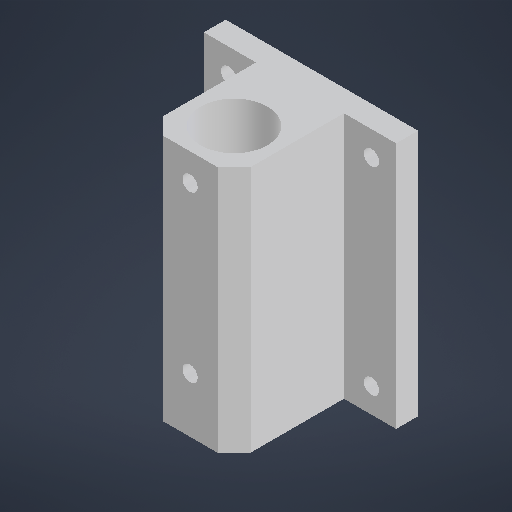
# Autodesk Inventor part: microscope mount
Saved by Autodesk Inventor 2026 (Build 300175050, 175E)
## iProperties
Created: 2025-07-01
Part Number: microscope mount
Material: Generic
Document SubType Name: Modeling
Designer: Tobymegacat
Density: 1 g/cm^3
Appearance: Default
Author: Tobymegacat
Autodesk Inventor part; units mm, degrees
ref_plane "YZ Plane" through (0, 0, 0) normal (1, 0, 0) x (0, 1, 0)
ref_plane "XZ Plane" through (0, 0, 0) normal (0, 1, 0) x (-1, 0, 0)
ref_plane "XY Plane" through (0, 0, 0) normal (0, 0, 1) x (1, 0, 0)
sketch "Sketch1" plane through (0, 0, 0) normal (0, 0, 1) x (1, 0, 0)
  line L0 (-16.3442, 35.2565) -> (18.6558, 35.2565)
  line L1 (18.6558, 35.2565) -> (18.6558, -9.7435)
  line L2 (18.6558, -9.7435) -> (-16.3442, -9.7435)
  line L3 (-16.3442, -9.7435) -> (-16.3442, 35.2565)
  point P0 (0, 0)
  dimension "d0" = 35
  dimension "d1" = 45
  constraints: 8 end point, 2 parallel, 1 horizontal, 1 perpendicular
  measures "d0" distance of L1.end L2.end
  measures "d1" distance between parallel lines of L0 L2
extrude "Extrusion1" add sketch "Sketch1" along normal blind 4
sketch "Sketch2" plane through (0, 0, 4) normal (0, 0, 1) x (1, 0, 0)
  line L0 (-6.8442, -9.7435) -> (9.1558, -9.7435)
  line L1 (9.1558, -9.7435) -> (9.1558, 35.2565)
  line L2 (9.1558, 35.2565) -> (-6.8442, 35.2565)
  line L3 (-6.8442, 35.2565) -> (-6.8442, -9.7435)
  line L4 (-16.3442, -9.7435) -> (18.6558, -9.7435) projected
  line L5 (18.6558, 35.2565) -> (-16.3442, 35.2565) projected
  line L6 (-6.8442, 14.4079) -> (-16.3442, 14.4079)
  line L7 (-16.3442, 35.2565) -> (-16.3442, -9.7435) projected
  line L8 (9.1558, 13.7437) -> (18.6558, 13.7437)
  line L9 (18.6558, -9.7435) -> (18.6558, 35.2565) projected
  point P0 (0, 0)
  dimension "d4" = 16
  constraints: 12 end point, 6 point on line, 3 horizontal, 3 parallel, 1 perpendicular
  measures "d4" distance of L1.end L2.end
extrude "Extrusion2" add sketch "Sketch2" along normal blind 20 contours L3 L2 L1 L0
sketch "Sketch3" plane through (-16.3442, 35.2565, 0) normal (0, 1, 0) x (1, 0, 0)
  circle A0 centre (17.5, -16) radius 6.1
  line L0 (25.5, -4) -> (25.5, -24) projected
  line L1 (25.5, -24) -> (9.5, -24) projected
  point P0 (16.3442, 0)
  dimension "d7" = 12.2
  dimension "d8" = 8
  dimension "d9" = 8
  constraints: 1 centre point
  measures "d7" diameter of A0
  measures "d8" distance from line of L0 A0.centre
  measures "d9" distance from line of L1 A0.centre
extrude "Extrusion3" cut sketch "Sketch3" against normal blind 45
chamfer "Chamfer1" distance 3 angle 45 2 edges at (-6.8442, 12.7565, 24) (9.1558, 12.7565, 24)
sketch "Sketch4" plane through (0, 0, 24) normal (0, 0, 1) x (1, 0, 0)
  line L0 (6.1558, 35.2565) -> (-3.8442, 35.2565) projected
  line L1 (6.1558, 35.2565) -> (6.1558, -9.7435) projected
  line L2 (-3.8442, -9.7435) -> (6.1558, -9.7435) projected
  point P0 (0, 0)
  point P1 (1.1558, 30.2565)
  point P2 (1.1558, 0.2565)
  dimension "d15" = 5
  dimension "d16" = 5
  dimension "d17" = 10
  dimension "d18" = 5
  measures "d15" distance from line of L0 point (1.156, 30.256)
  measures "d16" distance from line of L1 point (1.156, 30.256)
  measures "d17" distance from line of L2 point (1.156, 0.256)
  measures "d18" distance from line of L1 point (1.156, 0.256)
hole "Hole1" at (1.1558, 30.2565, 24) at (1.1558, 0.2565, 24) direction (0, 0, -1) diameter 2.8 depth 10
sketch "Sketch5" plane through (0, 0, 4) normal (0, 0, 1) x (1, 0, 0)
  line L0 (-6.8442, 35.2565) -> (-16.3442, 35.2565) projected
  line L1 (-16.3442, 35.2565) -> (-16.3442, -9.7435) projected
  point P0 (0, 0)
  point P1 (-11.8442, 30.7565)
  dimension "d26" = 4.5
  dimension "d27" = 4.5
  measures "d26" distance from line of L0 point (-11.844, 30.756)
  measures "d27" distance from line of L1 point (-11.844, 30.756)
hole "Hole2" at (-11.8442, 30.7565, 4) direction (0, 0, -1) diameter 2.8 depth 10
pattern_linear "Rectangular Pattern1" count 2 spacing 26 along (1, 0, 0) count 2 spacing 36 along (0, -1, 0) of "Hole2"
body "Solid1"
